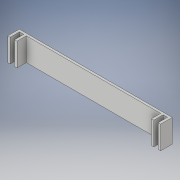
# Autodesk Inventor part: Potentiometer Carrier
Saved by Autodesk Inventor 2019 (Build 230136000, 136)
## iProperties
Created: 2019-01-04
Part Number: Potentiometer Carrier
Material: Generic
Document SubType Name: Modeling
Designer: Martin
Density: 1 g/cm^3
Appearance: Default
Author: Martin
Autodesk Inventor part; units mm, degrees
ref_plane "YZ Plane" through (0, 0, 0) normal (1, 0, 0) x (0, 1, 0)
ref_plane "XZ Plane" through (0, 0, 0) normal (0, 1, 0) x (-1, 0, 0)
ref_plane "XY Plane" through (0, 0, 0) normal (0, 0, 1) x (1, 0, 0)
sketch "Sketch1" plane through (0, 0, 0) normal (0, 0, 1) x (1, 0, 0)
  line L0 (-66, 10) -> (66, 10)
  line L1 (66, 10) -> (66, -10)
  line L2 (66, -10) -> (-66, -10)
  line L3 (-66, -10) -> (-66, 10)
  line L4 (-63.85, 10) -> (63.85, 10) construction
  line L5 (63.85, 10) -> (63.85, -10) construction
  line L6 (63.85, -10) -> (-63.85, -10) construction
  line L7 (-63.85, -10) -> (-63.85, 10) construction
  line L8 (-60.15, 10) -> (60.15, 10) construction
  line L9 (60.15, 10) -> (60.15, -10) construction
  line L10 (60.15, -10) -> (-60.15, -10) construction
  line L11 (-60.15, -10) -> (-60.15, 10) construction
  line L12 (-58, 10) -> (58, 10) construction
  line L13 (58, 10) -> (58, -10) construction
  line L14 (58, -10) -> (-58, -10) construction
  line L15 (-58, -10) -> (-58, 10) construction
  line L16 (-66, 10) -> (-63.85, 10)
  line L17 (-63.85, 10) -> (-63.85, -10)
  line L18 (-63.85, -10) -> (-66, -10)
  line L19 (-66, -10) -> (-66, 10)
  line L20 (-60.15, 10) -> (-58, 10)
  line L21 (-58, 10) -> (-58, -10)
  line L22 (-58, -10) -> (-60.15, -10)
  line L23 (-60.15, -10) -> (-60.15, 10)
  line L24 (58, 10) -> (60.15, 10)
  line L25 (60.15, 10) -> (60.15, -10)
  line L26 (60.15, -10) -> (58, -10)
  line L27 (58, -10) -> (58, 10)
  line L28 (63.85, 10) -> (66, 10)
  line L29 (66, 10) -> (66, -10)
  line L30 (66, -10) -> (63.85, -10)
  line L31 (63.85, -10) -> (63.85, 10)
  dimension "d0" = 132
  dimension "d7" = 20
  dimension "d10" = 2.15
  dimension "d11" = 8
  dimension "d12" = 2.15
  dimension "d13" = 8
  dimension "d14" = 2.15
  dimension "d15" = 2.15
  constraints: 64 end point, 16 parallel, 8 horizontal, 8 perpendicular
  measures "d0" distance of L1.end L2.end
  measures "d7" distance of L12.end L13.end
  measures "d10" distance between parallel lines of L17 L3
  measures "d11" distance between parallel lines of L15 L3
  measures "d12" distance between parallel lines of L11 L21
  measures "d13" distance between parallel lines of L13 L1
  measures "d14" distance between parallel lines of L1 L5
  measures "d15" distance between parallel lines of L9 L13
extrude "Extrusion1" add sketch "Sketch1" against normal blind 2
extrude "Extrusion2" add sketch "Sketch1" along normal blind 8 contours L0 L17 L2 L3 | L0 L21 L2 L23 | L0 L25 L2 L27 | L0 L1 L2 L31
body "Solid1"
